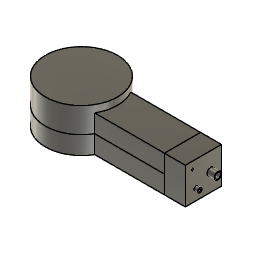
concept 1 housing v1 (Autodesk Fusion 360 design; units mm, degrees)
Autodesk Fusion 360 part; units mm, degrees
sketch "Sketch1" plane through (0, 0, 0) normal (0, 0, 1) x (1, 0, 0)
  line L0 (140, -25) -> (37.4166, -25)
  line L1 (140, 25) -> (37.4166, 25)
  arc A0 (43.3013, 25) -> (43.3013, -25) centre (0, 0) ccw
  arc A1 (39.7995, 25) -> (39.7995, -25) centre (0, 0) ccw
  line L2 (144, 0) -> (144, -19)
  line L3 (144, -19) -> (40.7922, -19)
  line L4 (140, -15) -> (42.4264, -15)
  line L5 (144, 0) -> (144, 19)
  line L6 (144, 19) -> (40.7922, 19)
  line L7 (140, 15) -> (42.4264, 15)
  arc A2 (42.4264, 15) -> (42.4264, -15) centre (0, 0) ccw
  line L8 (140, 25) -> (140, 19)
  line L9 (140, -19) -> (140, -25)
  line L10 (140, -15) -> (144, -15)
  line L11 (140, 15) -> (144, 15)
  line L12 (140, 19) -> (140, -19)
  dimension "d2" = 100
  dimension "d3" = 94
  dimension "d4" = 90
  dimension "d9" = 144
  dimension "d13" = 144
  constraint coincident A0.centre A1.centre
  constraint concentric A0 A1
  constraint concentric A0 A2
  constraint horizontal L0
  constraint horizontal L1
  constraint coincident L1 A0.start
  constraint coincident L1 A1.start
  constraint coincident L0 A0.end
  constraint coincident L0 A1.end
  constraint coincident L1.end A2
  constraint coincident L0.end A2
  constraint vertical L2
  constraint horizontal L3
  constraint horizontal L4
  constraint vertical L5
  constraint horizontal L6
  constraint horizontal L7
  constraint coincident L6.end A2
  constraint coincident L3.end A2
  constraint perpendicular L0 L8
  constraint collinear L8 L9
  constraint coincident L2 L10.end
  constraint perpendicular L2 L10
  constraint coincident L5 L11.end
  constraint perpendicular L5 L11
  constraint coincident L6 L8.end
  constraint coincident L3 L9.start
  constraint perpendicular L3 L12
  measures "d2" diameter of A0
  measures "d3" diameter of A1
  measures "d4" diameter of A2
  measures "d9" distance of A0.centre L2.start
  measures "d13" distance of A0.centre L2.start
extrude "Extrude1" add sketch "Sketch1" along normal blind 5 contours L4 L7 A2 L12 makes body 1
extrude "Extrude2" add sketch "Sketch1" along normal blind 27 contours L3 L4 A2 L12 bodies 1
extrude "Extrude3" add sketch "Sketch1" along normal blind 27 contours L2 L3 L10 L12 | L0 L1 A1 A2 | L5 L6 L11 L12 | L6 L7 A2 L12 bodies 1
extrude "Extrude4" add sketch "Sketch1" along normal blind 25 contours L0 L3 A2 L9 | L0 L1 A0 A1 | L1 L6 A2 L8 bodies 1
extrude "Extrude5" cut sketch "Sketch1" along normal blind 2 contours L2 L3 L10 L12 | L5 L6 L11 L12 bodies 1
extrude "Extrude6" add sketch "Sketch1" along normal blind 5 contours L2 L5 L10 L11 L12 bodies 1
extrude "Extrude7" cut sketch "Sketch1" along normal blind 2 contours L2 L5 L10 L11 L12 bodies 1
move_body "Move1" bodies 1 to x (1, 0, 0) y (0, 1, 0) z (0, 0, 1) at (0, 160, 0)
extrude "Extrude8" add sketch "Sketch1" along normal blind 25 separate body contours L0 L3 A2 L9 | L0 L1 A0 A1 | L3 L4 A2 L12 | L0 L1 A1 A2 | L1 L6 A2 L8 | L4 L7 A2 L12 | L6 L7 A2 L12 makes body 2
extrude "Extrude9" add sketch "Sketch1" along normal blind 23 contours L2 L3 L10 L12 | L2 L5 L10 L11 L12 | L5 L6 L11 L12 bodies 2
extrude "Extrude10" cut sketch "Sketch1" along normal blind 20 contours L4 L7 A2 L12 | L2 L5 L10 L11 L12 bodies 2
extrude "Extrude11" cut sketch "Sketch1" along normal blind 2 contours L2 L3 L10 L12 | L3 L4 A2 L12 | L0 L1 A1 A2 | L5 L6 L11 L12 | L6 L7 A2 L12 bodies 2
sketch "Sketch2" plane through (0, 0, 0) normal (0, 0, 1) x (1, 0, 0)
  circle A0 centre (0, 0) radius 50
  circle A1 centre (0, 0) radius 45
  dimension "d40" = 100
  dimension "d45" = 90
  constraint coincident A0.centre A1.centre
  measures "d40" diameter of A0
  measures "d45" diameter of A1
extrude "Extrude12" cut sketch "Sketch2" along normal blind 35 contours A0 | A1 bodies 2
extrude "Extrude13" add sketch "Sketch2" along normal blind 35 contours A0 | A1 bodies 2
extrude "Extrude14" cut sketch "Sketch2" along normal blind 25 contours A1 bodies 2
extrude "Extrude15" cut sketch "Sketch1" along normal blind 20 contours L4 L7 A2 L12 bodies 2
extrude "Extrude16" cut sketch "Sketch1" along normal blind 2 contours L0 L1 A1 A2 bodies 2
extrude "Extrude17" cut sketch "Sketch1" along normal blind 2 contours L3 L4 A2 L12 | L6 L7 A2 L12 bodies 2
move_body "Move2" bodies 1 2 to x (1, 0, 0) y (0, 1, 0) z (0, 0, 1) at (0, -80, 0)
extrude "Extrude18" add sketch "Sketch1" along normal blind 50 separate body contours L1 L6 A2 L8 makes body 3
extrude "Extrude19" add sketch "Sketch1" along normal blind 50 separate body contours L0 L3 A2 L9 | L2 L3 L10 L12 | L2 L5 L10 L11 L12 | L5 L6 L11 L12 makes body 4
extrude "Extrude20" add 1 faces at (140, -21, 16.6667) along direction (1, 0, 0) blind 4 on bodies 4 bodies 4
extrude "Extrude21" add 1 faces at (140, 23, 16.6667) along direction (1, 0, 0) blind 4 on bodies 3 bodies 3 4
extrude "Extrude22" cut sketch "Sketch1" along normal blind 50 contours L0 L3 A2 L9 bodies 3
extrude "Extrude23" cut sketch "Sketch1" along normal blind 50 contours L1 L6 A2 L8 bodies 3
extrude "Extrude24" add 1 faces at (144, 8.3333, 16.6667) along direction (1, 0, 0) blind 25 on bodies 3 bodies 3
extrude "Extrude25" cut sketch "Sketch1" along normal blind 48 contours L2 L3 L10 L12 | L2 L5 L10 L11 L12 | L5 L6 L11 L12 bodies 3
extrude "Extrude26" add sketch "Sketch1" along normal blind 2 contours L2 L3 L10 L12 | L2 L5 L10 L11 L12 | L5 L6 L11 L12 bodies 3
extrude "Extrude27" cut 1 faces at (144, -6.3333, 17.3333) along direction (1, 0, 0) blind 20 on bodies 3 bodies 3
extrude "Extrude28" cut 1 faces at (164, -6.3333, 17.3333) along direction (1, 0, 0) blind 3 on bodies 3 bodies 3
cylinder "CylinderPrimitive1" add diameter 10 height 15 placed x (0, 0, -1) y (0, 1, 0) z (1, 0, 0) at (169, 10, 25) bodies 3
cylinder "CylinderPrimitive2" cut diameter 8 height -155 placed x (0, 0, -1) y (0, 1, 0) z (1, 0, 0) at (184, 10, 25) bodies 3
extrude "Extrude29" cut 1 faces at (184, 9.5529, 20.3668) along direction (-1, 0, 0) blind 5 on bodies 3 bodies 3
cylinder "CylinderPrimitive3" cut diameter 3 height -10 placed x (0, 0, -1) y (0, 1, 0) z (1, 0, 0) at (169, -15, 40) bodies 3
cylinder "CylinderPrimitive4" add diameter 6 height 5 placed x (0, 0, -1) y (0, 1, 0) z (1, 0, 0) at (169, -10, 15) bodies 3
cylinder "CylinderPrimitive5" cut diameter 3 height -55555 placed x (0, 0, -1) y (0, 1, 0) z (1, 0, 0) at (174, -10, 15) bodies 3
move_body "Move3" bodies 3 to x (1, 0, 0) y (0, 1, 0) z (0, 0, 1) at (110, 0, 0)
move_body "Move4" bodies 2 1 to x (1, 0, 0) y (0, 1, 0) z (0, 0, 1) at (0, -80, 0)
move_body "Move5" bodies 2 to x (1, 0, 0) y (0, 1, 0) z (0, 0, 1) at (0, 160, 40)
move_body "Move6" bodies 3 to x (1, 0, 0) y (0, 1, 0) z (0, 0, 1) at (-90, 0, 0)
move_body "Move7" bodies 2 to x (1, 0, 0) y (0, 1, 0) z (0, 0, 1) at (0, 0, -10)
move_body "Move8" bodies 2 to x (1, 0, 0) y (0, 1, 0) z (0, 0, 1) at (0, 0, -5)
move_body "Move9" bodies 3 to x (1, 0, 0) y (0, 1, 0) z (0, 0, 1) at (-20, 0, 0)
equation "x = 100 mm"
equation "d2 = x"
equation "d3 = x - 6 mm"
equation "d4 = x - 10 mm"
equation "d9 = x + x / 2 - 6 mm"
equation "d13 = x + x / 2 - 6 mm"
equation "y = 25 mm"
equation "d20 = y + 2 mm"
equation "d22 = y + 2 mm"
equation "d24 = y"
equation "d32 = y"
equation "d34 = y - 2 mm"
equation "d36 = y - 5 mm"
equation "d40 = x"
equation "d41 = y + 10 mm"
equation "d43 = y + 10 mm"
equation "d45 = x - 10 mm"
equation "d46 = y"
equation "d48 = y - 5 mm"
equation "d54 = 2 * y"
equation "d56 = 2 * y"
equation "d62 = 2 * y"
equation "d64 = 2 * y"
equation "d66 = x / 4"
equation "d68 = y * 2 - 2 mm"
